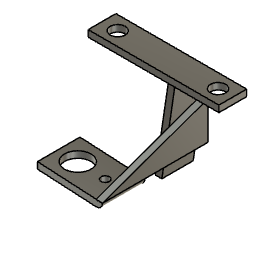
Assembly v15 (Autodesk Fusion 360 archive; units mm, degrees)
design "Mount"
Autodesk Fusion 360 part; units mm, degrees
sketch "Sketch4" plane through (0, 0, 0) normal (0, 0, 1) x (1, 0, 0)
  line L0 (-47.7, 10.125) -> (47.7, 10.125)
  line L1 (47.7, 10.125) -> (47.7, -10.125)
  line L2 (47.7, -10.125) -> (-47.7, -10.125)
  line L3 (-47.7, -10.125) -> (-47.7, 10.125)
  line L4 (-47.7, 0) -> (47.7, 0) construction
  circle A0 centre (36.95, 0) radius 5.5
  line L5 (0.3455, 47) -> (0.3455, -29) construction
  circle A1 centre (-36.2591, 0) radius 5.5
  line L6 (42.45, 3.7083) -> (42.45, -3.7083) construction
  point P0 (47.7, 0)
  point P1 (-47.7, 0)
  point P2 (42.45, 0)
  dimension "d16" = 95.4
  dimension "d17" = 20.25
  dimension "d18" = 11
  dimension "d20" = 5.25
  constraint perpendicular L0 L1
  constraint perpendicular L2 L3
  constraint parallel L0 L2
  constraint midpoint L1 P0
  constraint midpoint L3 P1
  constraint coincident P1 L4.start
  constraint coincident P0 L4.end
  constraint midpoint L4 origin
  constraint coincident L4 A0.centre
  constraint vertical L5
  constraint symmetric A0 L5 A1
  constraint coincident L4 P2
  constraint coincident A0 P2
  constraint midpoint L6 P2
  constraint tangent A0 L6
  measures "d16" distance of L1 L3
  measures "d17" distance of L0.start L2.end
  measures "d18" diameter of A0
  measures "d20" distance of L1 L6
extrude "Extrude2" add sketch "Sketch4" along normal blind 4.7625
sketch "Sketch5" plane through (0, 0, 0) normal (0, 0, -1) x (1, 0, 0)
  circle A0 centre (36.95, 0) radius 5.5
  circle A1 centre (-36.2591, 0) radius 5.5
  line L0 (47.7, 10.125) -> (-47.7, 10.125)
  line L1 (-47.7, 10.125) -> (-47.7, -10.125)
  line L2 (-47.7, -10.125) -> (47.7, -10.125)
  line L3 (47.7, -10.125) -> (47.7, 10.125)
  line L4 (10.7, 15.5999) -> (15.4625, 15.5999)
  line L5 (15.4625, 15.5999) -> (15.4625, -14.8215)
  line L6 (10.7, -14.8215) -> (10.7, 15.5999)
  line L7 (10.7, -14.8215) -> (15.4625, -14.8215)
  dimension "d24" = 37
  dimension "d25" = 4.7625
  constraint horizontal L4
  constraint vertical L5
  constraint vertical L6
  constraint coincident L4.start L6.end
  constraint coincident L5.end L7.end
  constraint coincident L6.start L7.start
  constraint horizontal L7
  measures "d24" distance of L3 L6
  measures "d25" distance of L5 L6
extrude "Extrude3" add sketch "Sketch5" along normal blind 53.2375 contours L0 L2 L5 L6 | L0 L4 L5 L6 | L2 L5 L6 L7
sketch "Sketch6" plane through (15.4625, 0, 0) normal (1, 0, 0) x (0, 1, 0)
  line L0 (-10.125, 0) -> (-15.5999, 0)
  line L1 (-15.5999, 0) -> (-15.5999, -53.2375)
  line L2 (-15.5999, -53.2375) -> (14.8215, -53.2375)
  line L3 (14.8215, -53.2375) -> (14.8215, 0)
  line L4 (14.8215, 0) -> (10.125, 0)
  line L5 (10.125, 0) -> (-10.125, 0)
  line L6 (-10.125, 0) -> (10.125, 0)
  line L7 (10.125, 0) -> (10.125, -15)
  line L8 (-10.125, 0) -> (-19.5122, -53.2375)
  line L9 (10.125, -15) -> (3.3827, -53.2375)
  line L10 (-19.5122, -53.2375) -> (3.3827, -53.2375)
  point P0 (10.125, 0)
  dimension "d30" = 100
  constraint horizontal L6
  constraint vertical L7
  constraint coincident L0.start L5.end
  constraint coincident P0 L4.end
  constraint parallel L8 L9
  constraint coincident L7.end L9.start
  constraint horizontal L10
  constraint collinear L2 L10
  measures "d30" angle of L6 L8
extrude "Extrude4" cut sketch "Sketch6" against normal up to surface (4.7625 mm away) contours L0 L1 L8 | L2 L3 L4 L7 L9
extrude "Extrude5" add sketch "Sketch6" against normal up to surface (4.7625 mm away) contours L1 L8 L10
sketch "Sketch7" plane through (15.4625, 0, 0) normal (1, 0, 0) x (0, 1, 0)
  line L0 (3.3827, -53.2375) -> (10.125, -15)
  line L1 (10.125, -15) -> (10.125, 0)
  line L2 (10.125, 0) -> (-10.125, 0)
  line L3 (-10.125, 0) -> (-19.5122, -53.2375)
  line L4 (-19.5122, -53.2375) -> (3.3827, -53.2375)
  line L5 (-67.6425, -42.2375) -> (9.3575, -14.7375)
  line L6 (9.3575, -14.7375) -> (9.3575, -42.2375)
  line L7 (9.3575, -42.2375) -> (-67.6425, -42.2375)
  line L8 (-10.125, 4.7625) -> (10.125, 4.7625)
  dimension "d35" = 77
  dimension "d36" = 27.5
  dimension "d37" = 47
  constraint horizontal L7
  constraint perpendicular L6 L7
  measures "d35" distance of L5.start L6.end
  measures "d36" distance of L5.end L6.end
  measures "d37" distance of L7 L8
extrude "Extrude6" add sketch "Sketch7" along normal blind 4.7625 contours L0 L3 L5 L6 L7 | L0 L6 L7 | L3 L5 L7
sketch "Sketch8" plane through (0, 0, -42.2375) normal (0, 0, -1) x (1, 0, 0)
  line L0 (15.4625, -5.3223) -> (15.4625, -9.3575)
  line L1 (15.4625, -9.3575) -> (20.225, -9.3575)
  line L2 (20.225, -9.3575) -> (20.225, 67.6425)
  line L3 (20.225, 67.6425) -> (15.4625, 67.6425)
  line L4 (15.4625, 67.6425) -> (15.4625, 17.5726)
  line L5 (15.4625, 17.5726) -> (15.4625, -5.3223)
  line L6 (20.225, 67.6425) -> (-29.775, 65.0221)
  line L7 (-29.775, 65.0221) -> (-29.775, 34.0221)
  line L8 (-29.775, 34.0221) -> (20.225, 36.6425)
  line L9 (20.225, 36.6425) -> (20.225, 67.6425)
  circle A0 centre (-15.125, 50.2899) radius 9.65
  line L10 (-15.125, 40.6399) -> (-15.125, 59.9399) construction
  line L11 (-5.475, 50.2899) -> (-24.775, 50.2899) construction
  line L12 (-24.775, 58.5104) -> (-24.775, 42.0694) construction
  line L13 (-15.1316, 59.9399) -> (-15.1184, 59.9399) construction
  line L14 (-15.1316, 40.6399) -> (-15.1184, 40.6399) construction
  line L15 (-15.9351, 65.7475) -> (-14.3149, 34.8324) construction
  line L16 (15.4625, 51.8929) -> (-29.775, 49.5221) construction
  circle A1 centre (5.996, 51.3968) radius 3
  line L17 (-5.6407, 53.7042) -> (-5.3358, 47.8857) construction
  line L18 (2.8046, 54.9702) -> (3.1956, 47.5094) construction
  point P0 (-15.125, 50.2899)
  point P1 (-5.4882, 50.795)
  point P2 (3.0001, 51.2398)
  dimension "d40" = 3
  dimension "d41" = 50
  dimension "d42" = 31
  dimension "d44" = 19.3
  dimension "d45" = 5
  dimension "d47" = 30.9575
  dimension "d49" = 6
  dimension "d50" = 8.5
  constraint vertical L7
  constraint coincident L2.end L3.start
  constraint parallel L6 L8
  constraint parallel L2 L9
  constraint midpoint P0 L11
  constraint midpoint P0 L10
  constraint horizontal L11
  constraint vertical L10
  constraint coincident A0 L11.start
  constraint coincident A0 L10.start
  constraint midpoint L11.end L12
  constraint tangent A0 L12
  constraint midpoint L10.end L13
  constraint tangent A0 L13
  constraint symmetric L11 L13.start L14.start
  constraint symmetric L11 L13.end L14.end
  constraint perpendicular L6 L15
  constraint coincident L6 L15.start
  constraint coincident L8 L15.end
  constraint perpendicular L15 L16
  constraint coincident L7 L16.end
  constraint coincident L4 L16.start
  constraint midpoint L15 P0
  constraint coincident L16 P0
  constraint coincident P0 A0.centre
  constraint coincident L16 A1.centre
  constraint coincident A0 P1
  constraint coincident L16 P1
  constraint midpoint L17 P1
  constraint tangent A0 L17
  constraint coincident L16 P2
  constraint coincident A1 P2
  constraint midpoint L18 P2
  constraint tangent A1 L18
  measures "d40" angle of L3 L6
  measures "d41" distance of L7 L9
  measures "d42" distance of L6.end L7.end
  measures "d44" diameter of A0
  measures "d45" distance of L7 L12
  measures "d47" distance of L6 L8
  measures "d49" diameter of A1
  measures "d50" distance of L17 L18
extrude "Extrude7" add sketch "Sketch8" along normal blind 4.7625 contours L4 L6 L7 L8 | L2 L4 L6 L8 L9
fillet "Fillet1" radius 4.7625 1 edges at (20.225, -52.1425, -47)
equation "d21 = ( 3 / 16 ) * 1 in"
equation "d25 = ( 3 / 16 ) * 1 in"
equation "d26 = 58 mm - ( ( 3 / 16 ) * 1 in )"
equation "d30 = 90 deg + 10 deg"
equation "d38 = ( 3 / 16 ) * 1 in"
equation "d51 = ( 3 / 16 ) * 1 in"
equation "d54 = ( 3 / 16 ) * 1 in"

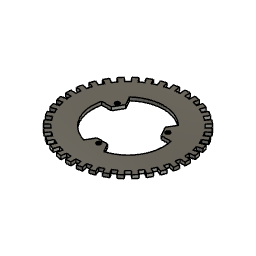
design "Trigger Wheel (Final)"
Autodesk Fusion 360 part; units mm, degrees
sketch "FrontOn" plane through (0, 0, 0) normal (0, 0, 1) x (1, 0, 0)
  line L0 (3.7212, -85.2299) -> (-3.7212, -85.2299)
  line L1 (3.7212, -85.2299) -> (3.393, -77.7135)
  line L2 (-3.7212, -85.2299) -> (-3.393, -77.7135)
  line L3 (18.4647, -83.2889) -> (11.1353, -84.5813)
  line L4 (18.4647, -83.2889) -> (16.8363, -75.9436)
  line L5 (11.1353, -84.5813) -> (10.1533, -77.122)
  line L6 (32.6472, -78.8172) -> (25.6536, -81.3627)
  line L7 (32.6472, -78.8172) -> (29.768, -71.8663)
  line L8 (25.6536, -81.3627) -> (23.3912, -74.1873)
  line L9 (45.8376, -71.9507) -> (39.3923, -75.6719)
  line L10 (45.8376, -71.9507) -> (41.7952, -65.6053)
  line L11 (39.3923, -75.6719) -> (35.9183, -68.9984)
  line L12 (57.6354, -62.898) -> (51.9341, -67.6819)
  line L13 (57.6354, -62.898) -> (52.5525, -57.351)
  line L14 (51.9341, -67.6819) -> (47.354, -61.713)
  line L15 (67.6819, -51.9341) -> (62.898, -57.6354)
  line L16 (67.6819, -51.9341) -> (61.713, -47.354)
  line L17 (62.898, -57.6354) -> (57.351, -52.5525)
  line L18 (75.6719, -39.3923) -> (71.9507, -45.8376)
  line L19 (75.6719, -39.3923) -> (68.9984, -35.9183)
  line L20 (71.9507, -45.8376) -> (65.6053, -41.7952)
  line L21 (81.3627, -25.6536) -> (78.8172, -32.6472)
  line L22 (81.3627, -25.6536) -> (74.1873, -23.3912)
  line L23 (78.8172, -32.6472) -> (71.8663, -29.768)
  line L24 (84.5813, -11.1353) -> (83.2889, -18.4647)
  line L25 (84.5813, -11.1353) -> (77.122, -10.1533)
  line L26 (83.2889, -18.4647) -> (75.9436, -16.8363)
  line L27 (85.2299, 3.7212) -> (85.2299, -3.7212)
  line L28 (85.2299, 3.7212) -> (77.7135, 3.393)
  line L29 (85.2299, -3.7212) -> (77.7135, -3.393)
  line L30 (83.2889, 18.4647) -> (84.5813, 11.1353)
  line L31 (83.2889, 18.4647) -> (75.9436, 16.8363)
  line L32 (84.5813, 11.1353) -> (77.122, 10.1533)
  line L33 (78.8172, 32.6472) -> (81.3627, 25.6536)
  line L34 (78.8172, 32.6472) -> (71.8663, 29.768)
  line L35 (81.3627, 25.6536) -> (74.1873, 23.3912)
  line L36 (71.9507, 45.8376) -> (75.6719, 39.3923)
  line L37 (71.9507, 45.8376) -> (65.6053, 41.7952)
  line L38 (75.6719, 39.3923) -> (68.9984, 35.9183)
  line L39 (62.898, 57.6354) -> (67.6819, 51.9341)
  line L40 (62.898, 57.6354) -> (57.351, 52.5525)
  line L41 (67.6819, 51.9341) -> (61.713, 47.354)
  line L42 (51.9341, 67.6819) -> (57.6354, 62.898)
  line L43 (51.9341, 67.6819) -> (47.354, 61.713)
  line L44 (57.6354, 62.898) -> (52.5525, 57.351)
  line L45 (39.3923, 75.6719) -> (45.8376, 71.9507)
  line L46 (39.3923, 75.6719) -> (35.9183, 68.9984)
  line L47 (45.8376, 71.9507) -> (41.7952, 65.6053)
  line L48 (25.6536, 81.3627) -> (32.6472, 78.8172)
  line L49 (25.6536, 81.3627) -> (23.3912, 74.1873)
  line L50 (32.6472, 78.8172) -> (29.768, 71.8663)
  line L51 (11.1353, 84.5813) -> (18.4647, 83.2889)
  line L52 (11.1353, 84.5813) -> (10.1533, 77.122)
  line L53 (18.4647, 83.2889) -> (16.8363, 75.9436)
  line L54 (-3.7212, 85.2299) -> (3.7212, 85.2299)
  line L55 (-3.7212, 85.2299) -> (-3.393, 77.7135)
  line L56 (3.7212, 85.2299) -> (3.393, 77.7135)
  line L57 (-18.4647, 83.2889) -> (-11.1353, 84.5813)
  line L58 (-18.4647, 83.2889) -> (-16.8363, 75.9436)
  line L59 (-11.1353, 84.5813) -> (-10.1533, 77.122)
  line L60 (-32.6472, 78.8172) -> (-25.6536, 81.3627)
  line L61 (-32.6472, 78.8172) -> (-29.768, 71.8663)
  line L62 (-25.6536, 81.3627) -> (-23.3912, 74.1873)
  line L63 (-45.8376, 71.9507) -> (-39.3923, 75.6719)
  line L64 (-45.8376, 71.9507) -> (-41.7952, 65.6053)
  line L65 (-39.3923, 75.6719) -> (-35.9183, 68.9984)
  line L66 (-57.6354, 62.898) -> (-51.9341, 67.6819)
  line L67 (-57.6354, 62.898) -> (-52.5525, 57.351)
  line L68 (-51.9341, 67.6819) -> (-47.354, 61.713)
  line L69 (-67.6819, 51.9341) -> (-62.898, 57.6354)
  line L70 (-67.6819, 51.9341) -> (-61.713, 47.354)
  line L71 (-62.898, 57.6354) -> (-57.351, 52.5525)
  line L72 (-75.6719, 39.3923) -> (-71.9507, 45.8376)
  line L73 (-75.6719, 39.3923) -> (-68.9984, 35.9183)
  line L74 (-71.9507, 45.8376) -> (-65.6053, 41.7952)
  line L75 (-81.3627, 25.6536) -> (-78.8172, 32.6472)
  line L76 (-81.3627, 25.6536) -> (-74.1873, 23.3912)
  line L77 (-78.8172, 32.6472) -> (-71.8663, 29.768)
  line L78 (-84.5813, 11.1353) -> (-83.2889, 18.4647)
  line L79 (-84.5813, 11.1353) -> (-77.122, 10.1533)
  line L80 (-83.2889, 18.4647) -> (-75.9436, 16.8363)
  line L81 (-85.2299, -3.7212) -> (-85.2299, 3.7212)
  line L82 (-85.2299, -3.7212) -> (-77.7135, -3.393)
  line L83 (-85.2299, 3.7212) -> (-77.7135, 3.393)
  line L84 (-83.2889, -18.4647) -> (-84.5813, -11.1353)
  line L85 (-83.2889, -18.4647) -> (-75.9436, -16.8363)
  line L86 (-84.5813, -11.1353) -> (-77.122, -10.1533)
  line L87 (-78.8172, -32.6472) -> (-81.3627, -25.6536)
  line L88 (-78.8172, -32.6472) -> (-71.8663, -29.768)
  line L89 (-81.3627, -25.6536) -> (-74.1873, -23.3912)
  line L90 (-71.9507, -45.8376) -> (-75.6719, -39.3923)
  line L91 (-71.9507, -45.8376) -> (-65.6053, -41.7952)
  line L92 (-75.6719, -39.3923) -> (-68.9984, -35.9183)
  line L93 (-62.898, -57.6354) -> (-67.6819, -51.9341)
  line L94 (-62.898, -57.6354) -> (-57.351, -52.5525)
  line L95 (-67.6819, -51.9341) -> (-61.713, -47.354)
  line L96 (-51.9341, -67.6819) -> (-57.6354, -62.898)
  line L97 (-51.9341, -67.6819) -> (-47.354, -61.713)
  line L98 (-57.6354, -62.898) -> (-52.5525, -57.351)
  line L99 (-39.3923, -75.6719) -> (-45.8376, -71.9507)
  line L100 (-39.3923, -75.6719) -> (-35.9183, -68.9984)
  line L101 (-45.8376, -71.9507) -> (-41.7952, -65.6053)
  line L102 (-25.6536, -81.3627) -> (-32.6472, -78.8172)
  line L103 (-25.6536, -81.3627) -> (-23.3912, -74.1873)
  line L104 (-32.6472, -78.8172) -> (-29.768, -71.8663)
  line L105 (-11.1353, -84.5813) -> (-18.4647, -83.2889)
  line L106 (-11.1353, -84.5813) -> (-10.1533, -77.122)
  line L107 (-18.4647, -83.2889) -> (-16.8363, -75.9436)
  line L108 (0, -70.9949) -> (0, -77.7875) construction
  arc A0 (3.393, -77.7135) -> (10.1533, -77.122) centre (0, 0) ccw
  arc A1 (-10.1533, -77.122) -> (-3.393, -77.7135) centre (0, 0) ccw
  arc A2 (-23.3912, -74.1873) -> (-16.8363, -75.9436) centre (0, 0) ccw
  arc A3 (-35.9183, -68.9984) -> (-29.768, -71.8663) centre (0, 0) ccw
  arc A4 (-47.354, -61.713) -> (-41.7952, -65.6053) centre (0, 0) ccw
  arc A5 (-57.351, -52.5525) -> (-52.5525, -57.351) centre (0, 0) ccw
  arc A6 (-65.6053, -41.7952) -> (-61.713, -47.354) centre (0, 0) ccw
  arc A7 (-71.8663, -29.768) -> (-68.9984, -35.9183) centre (0, 0) ccw
  arc A8 (-75.9436, -16.8363) -> (-74.1873, -23.3912) centre (0, 0) ccw
  arc A9 (-77.7135, -3.393) -> (-77.122, -10.1533) centre (0, 0) ccw
  arc A10 (-77.122, 10.1533) -> (-77.7135, 3.393) centre (0, 0) ccw
  arc A11 (-74.1873, 23.3912) -> (-75.9436, 16.8363) centre (0, 0) ccw
  arc A12 (-68.9984, 35.9183) -> (-71.8663, 29.768) centre (0, 0) ccw
  arc A13 (-61.713, 47.354) -> (-65.6053, 41.7952) centre (0, 0) ccw
  arc A14 (-52.5525, 57.351) -> (-57.351, 52.5525) centre (0, 0) ccw
  arc A15 (-41.7952, 65.6053) -> (-47.354, 61.713) centre (0, 0) ccw
  arc A16 (-29.768, 71.8663) -> (-35.9183, 68.9984) centre (0, 0) ccw
  arc A17 (-16.8363, 75.9436) -> (-23.3912, 74.1873) centre (0, 0) ccw
  arc A18 (-3.393, 77.7135) -> (-10.1533, 77.122) centre (0, 0) ccw
  arc A19 (10.1533, 77.122) -> (3.393, 77.7135) centre (0, 0) ccw
  arc A20 (23.3912, 74.1873) -> (16.8363, 75.9436) centre (0, 0) ccw
  arc A21 (35.9183, 68.9984) -> (29.768, 71.8663) centre (0, 0) ccw
  arc A22 (57.351, 52.5525) -> (52.5525, 57.351) centre (0, 0) ccw
  arc A23 (47.354, 61.713) -> (41.7952, 65.6053) centre (0, 0) ccw
  arc A24 (65.6053, 41.7952) -> (61.713, 47.354) centre (0, 0) ccw
  arc A25 (71.8663, 29.768) -> (68.9984, 35.9183) centre (0, 0) ccw
  arc A26 (75.9436, 16.8363) -> (74.1873, 23.3912) centre (0, 0) ccw
  arc A27 (77.7135, 3.393) -> (77.122, 10.1533) centre (0, 0) ccw
  arc A28 (77.122, -10.1533) -> (77.7135, -3.393) centre (0, 0) ccw
  arc A29 (74.1873, -23.3912) -> (75.9436, -16.8363) centre (0, 0) ccw
  arc A30 (68.9984, -35.9183) -> (71.8663, -29.768) centre (0, 0) ccw
  arc A31 (61.713, -47.354) -> (65.6053, -41.7952) centre (0, 0) ccw
  arc A32 (52.5525, -57.351) -> (57.351, -52.5525) centre (0, 0) ccw
  arc A33 (41.7952, -65.6053) -> (47.354, -61.713) centre (0, 0) ccw
  arc A34 (16.8363, -75.9436) -> (23.3912, -74.1873) centre (0, 0) ccw
  arc A35 (29.768, -71.8663) -> (35.9183, -68.9984) centre (0, 0) ccw
  circle A36 centre (0, 0) radius 50.8
  line L109 (14.4449, -48.703) -> (7.5367, -36.7378)
  line L110 (0, -105.8478) -> (0, 0) construction
  line L111 (-14.4449, -48.703) -> (-7.5367, -36.7378)
  line L112 (7.5367, -36.7378) -> (-7.5367, -36.7378)
  circle A37 centre (0, -41.7771) radius 2
  line L113 (34.9556, 36.8611) -> (28.0475, 24.8959)
  circle A38 centre (36.18, 20.8886) radius 2
  line L114 (28.0475, 24.8959) -> (35.5843, 11.8419)
  line L115 (49.4005, 11.8419) -> (35.5843, 11.8419)
  line L116 (-49.4005, 11.8419) -> (-35.5843, 11.8419)
  circle A39 centre (-36.18, 20.8886) radius 2
  line L117 (-35.5843, 11.8419) -> (-28.0475, 24.8959)
  line L118 (-34.9556, 36.8611) -> (-28.0475, 24.8959)
  circle A40 centre (0, 0) radius 41.7771 construction
  dimension "d36" = 85.2299
  dimension "d37" = 5
  dimension "d39" = 2.5
  dimension "d41" = 7.4424
  dimension "d43" = 360
  dimension "d63" = 101.6
  dimension "d64" = 120
  dimension "d65" = 4
  dimension "d66" = 77.7875
  dimension "d68" = 360
  dimension "d69" = 83.5542
  constraint horizontal L0
  constraint vertical L108
  constraint coincident L108.end A34
  constraint concentric A0 A34
  constraint concentric A1 A34
  constraint concentric A2 A34
  constraint concentric A3 A34
  constraint concentric A4 A34
  constraint concentric A5 A34
  constraint concentric A6 A34
  constraint concentric A7 A34
  constraint concentric A8 A34
  constraint concentric A9 A34
  constraint concentric A10 A34
  constraint concentric A11 A34
  constraint concentric A12 A34
  constraint concentric A13 A34
  constraint concentric A14 A34
  constraint concentric A15 A34
  constraint concentric A16 A34
  constraint concentric A17 A34
  constraint concentric A18 A34
  constraint concentric A19 A34
  constraint concentric A20 A34
  constraint concentric A21 A34
  constraint concentric A22 A34
  constraint concentric A22 A23
  constraint concentric A24 A34
  constraint concentric A25 A34
  constraint concentric A26 A34
  constraint concentric A27 A34
  constraint concentric A28 A34
  constraint concentric A29 A34
  constraint concentric A30 A34
  constraint concentric A31 A34
  constraint concentric A32 A34
  constraint concentric A33 A34
  constraint concentric A34 A35
  constraint concentric A29 A36
  constraint coincident A0.centre A1.centre
  constraint coincident A36 L109.start
  constraint symmetric L109.start L110 L111.start
  constraint symmetric L109.end L110 L111.end
  constraint coincident L110 A37.centre
  constraint vertical L110
  constraint concentric A35 A40
  constraint coincident A39.centre A40
  measures "d36" distance of A0.centre L0
  measures "d37" angle of L1 L2
  measures "d39" angle of L1 L108
  measures "d41" distance of L0.start L0.end
  measures "d63" diameter of A36
  measures "d64" angle of L109 L112
  measures "d65" diameter of A37
  measures "d66" radius of A34
  measures "d69" diameter of A40
extrude "Extrude4" add sketch "FrontOn" along normal blind 4.7625 contours L0 L1 L2 L3 L4 L5 L6 L7 L8 L9 L10 L11 L12 L13 L14 L15 L16 L17 L18 L19 L20 L21 L22 L23 L24 L25 L26 L27 L28 L29 L30 L31 L32 L33 L34 L35 L36 L37 L38 L39 L40 L41 L42 L43 L44 L45 L46 L47 L48 L49 L50 L51 L52 L53 L54 L55 L56 L57 L58 L59 L60 L61 L62 L63 L64 L65 L66 L67 L68 L69 L70 L71 L72 L73 L74 L75 L76 L77 L78 L79 L80 L81 L82 L83 L84 L85 L86 L87 L88 L89 L90 L91 L92 L93 L94 L95 L96 L97 L98 L99 L100 L101 L102 L103 L104 L105 L106 L107 A0 A1 A2 A3 A4 A5 A6 A7 A8 A9 A10 A11 A12 A13 A14 A15 A16 A17 A18 A19 A20 A21 A22 A23 A24 A25 A26 A27 A28 A29 A30 A31 A32 A33 A34 A35 | A36 L113 L114 L115 | A36 L109 L111 L112 | A36 L116 L117 L118
thread "Thread1" "ANSI Metric M Profile 6.0 M6x1 6H" major diameter 6.147 minor diameter 5.035 pitch 1 angle 60 modelled right hand crest width 0.2748 on face at (-34.1825, 20.7889, 3.175) crest through (-33.6625, 20.8886, 0.25) on face at (1.9975, -41.8768, 3.175) crest through (2.5175, -41.7771, 0.25) on face at (38.1776, 20.7889, 3.175) crest through (38.6975, 20.8886, 0.25)
equation "d25 = ( 360 / 36 / 2 ) * 1 deg"
equation "d36 = ( ( 6.125 / 2 ) * 1 in ) + d41"
equation "d37 = ( 360 / teeth / 2 ) * 1 deg"
equation "teeth = 36"
equation "d39 = d37 / 2"
equation "d42 = teeth"
equation "d61 = ( 3 / 16 ) * 1 in"
equation "d66 = ( 6.125 / 2 ) * 1 in"

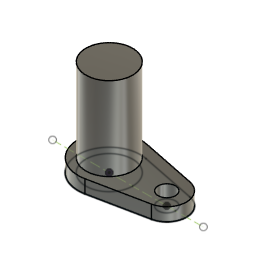
design "Hall Sensor"
Autodesk Fusion 360 part; units mm, degrees
sketch "Sketch1" plane through (0, 0, 0) normal (0, 0, 1) x (1, 0, 0)
  circle A0 centre (22, 0) radius 3.3
  line L0 (2.38, 11.6596) -> (23.5, 7.3485)
  line L1 (36, 0) -> (-21.665, 0) construction
  line L2 (2.38, -11.6596) -> (23.5, -7.3485)
  arc A1 (23.5, -7.3485) -> (23.5, 7.3485) centre (22, 0) ccw
  arc A2 (2.38, 11.6596) -> (2.38, -11.6596) centre (0, 0) ccw
  circle A3 centre (0, 0) radius 8.93
  dimension "d1" = 23.8
  dimension "d2" = 15
  dimension "d3" = 22
  dimension "d4" = 6.6
  dimension "d5" = 17.86
  constraint coincident A2.centre A3.centre
  constraint concentric A0 A1
  constraint tangent L0 A2
  constraint horizontal L1
  constraint coincident A0.centre L1
  constraint tangent L0 A1
  constraint tangent L2 A2
  constraint tangent L2 A1
  measures "d1" diameter of A2
  measures "d2" diameter of A1
  measures "d3" distance of A2.centre A0.centre
  measures "d4" diameter of A0
  measures "d5" diameter of A3
extrude "Extrude1" add sketch "Sketch1" along normal blind 5
extrude "Extrude2" add sketch "Sketch1" along normal blind 36.75 contours A3
equation "d8 = 5 mm + 31.75 mm"
